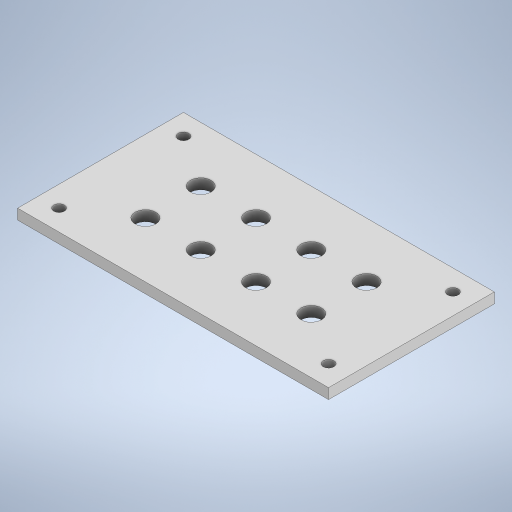
# Autodesk Inventor part: SequenceMachine_VialPlate
Saved by Autodesk Inventor 2023 (Build 270158000, 158)
## iProperties
Created: 2022-07-18
Part Number: SequenceMachine_VialPlate
Material: Generic
Document SubType Name: Modeling
Designer: devon
Density: 1 g/cm^3
Appearance: Default
Author: devon
Autodesk Inventor part; units mm, degrees
ref_plane "YZ Plane" through (0, 0, 0) normal (1, 0, 0) x (0, 1, 0)
ref_plane "XZ Plane" through (0, 0, 0) normal (0, 1, 0) x (-1, 0, 0)
ref_plane "XY Plane" through (0, 0, 0) normal (0, 0, 1) x (1, 0, 0)
sketch "Sketch1" plane through (0, 0, 0) normal (0, 1, 0) x (-1, 0, 0)
  circle A0 centre (0, 0) radius 6.35
  line L0 (0, 0) -> (0, 25.4) construction
  line L1 (0, 0) -> (-101.6, 0) construction
  line L2 (44.45, -33.8667) -> (-146.05, -33.8667)
  line L3 (-146.05, -33.8667) -> (-146.05, 67.7333)
  line L4 (-146.05, 67.7333) -> (44.45, 67.7333)
  line L5 (44.45, 67.7333) -> (44.45, -33.8667)
  circle A1 centre (31.75, -21.1667) radius 3.302
  circle A2 centre (-133.35, -21.1667) radius 3.302
  circle A3 centre (-133.35, 55.0333) radius 3.302
  circle A4 centre (31.75, 55.0333) radius 3.302
  circle A5 centre (-33.8667, 0) radius 6.35
  circle A6 centre (-67.7333, 0) radius 6.35
  circle A7 centre (-101.6, 0) radius 6.35
  circle A8 centre (0, 33.8667) radius 6.35
  circle A9 centre (-33.8667, 33.8667) radius 6.35
  circle A10 centre (-67.7333, 33.8667) radius 6.35
  circle A11 centre (-101.6, 33.8667) radius 6.35
  dimension "d0" = 12.7
  dimension "d15" = 6.604
  dimension "d16" = 12.7
  dimension "d17" = 12.7
  dimension "d18" = 6.604
  dimension "d19" = 12.7
  dimension "d20" = 6.604
  dimension "d21" = 12.7
  dimension "d22" = 6.604
  dimension "d25" = 101.6
  dimension "d26" = 33.8667
  dimension "d27" = 12.7
  dimension "d28" = 12.7
  dimension "d29" = 12.7
  dimension "d30" = 44.45
  dimension "d31" = 190.5
  dimension "d34" = 33.8667
  dimension "d37" = 33.8667
  constraints: 12 centre point, 12 end point, 2 horizontal, 2 parallel, 2 vertical, 1 coincident, 1 perpendicular, 14 other
  measures "d0" diameter of A0
  measures "d15" diameter of A1
  measures "d16" distance from line of L2 A1.centre
  measures "d17" distance from line of L5 A1.centre
  measures "d18" diameter of A2
  measures "d19" distance from line of L3 A2.centre
  measures "d20" diameter of A3
  measures "d21" distance from line of L4 A3.centre
  measures "d22" diameter of A4
  measures "d25" distance of L2.end L3.end
  measures "d26" distance from line of L2 point (0, 0)
  measures "d27" distance from line of L4 A4.centre
  measures "d28" distance from line of L5 A4.centre
  measures "d29" distance from line of L2 A2.centre
  measures "d30" distance from line of L5 point (0, 0)
  measures "d31" distance of L2.start L2.end
  measures "d34" distance of L0.start A5.centre
  measures "d37" distance of L0.start A8.centre
extrude "Extrusion2" add sketch "Sketch1" along normal blind 6.35
equation "\"d26\" = 0.333333 * d25"
equation "\"d37\" = 0.333333 * d25"
body "Solid2"
